Autodesk Fusion 360 part; units mm, degrees
(part 21 of 40)
  line L2220 (15.7293, 63.975) -> (15.8242, 64.105) construction
  line L2221 (15.8242, 64.105) -> (15.92, 64.2346) construction
  line L2222 (15.92, 64.2346) -> (16.0168, 64.3638) construction
  line L2223 (16.0168, 64.3638) -> (16.1146, 64.4926) construction
  line L2224 (16.1146, 64.4926) -> (16.2132, 64.6209) construction
  line L2225 (16.2132, 64.6209) -> (16.3127, 64.7488) construction
  line L2226 (16.3127, 64.7488) -> (16.4131, 64.8762) construction
  line L2227 (16.4131, 64.8762) -> (16.5144, 65.0032) construction
  line L2228 (16.5144, 65.0032) -> (16.6166, 65.1298) construction
  line L2229 (16.6166, 65.1298) -> (16.7196, 65.256) construction
  line L2230 (16.7196, 65.256) -> (16.8235, 65.3817) construction
  line L2231 (16.8235, 65.3817) -> (16.9283, 65.507) construction
  line L2232 (16.9283, 65.507) -> (17.0338, 65.6318) construction
  line L2233 (17.0338, 65.6318) -> (17.1402, 65.7562) construction
  line L2234 (17.1402, 65.7562) -> (17.2474, 65.8802) construction
  line L2235 (17.2474, 65.8802) -> (17.3555, 66.0038) construction
  line L2236 (17.3555, 66.0038) -> (17.4643, 66.1269) construction
  line L2237 (17.4643, 66.1269) -> (17.5739, 66.2497) construction
  line L2238 (17.5739, 66.2497) -> (17.6842, 66.3719) construction
  line L2239 (17.6842, 66.3719) -> (17.7954, 66.4938) construction
  line L2240 (17.7954, 66.4938) -> (17.9073, 66.6152) construction
  line L2241 (17.9073, 66.6152) -> (18.02, 66.7362) construction
  line L2242 (18.02, 66.7362) -> (18.1335, 66.8568) construction
  line L2243 (18.1335, 66.8568) -> (18.2477, 66.9769) construction
  line L2244 (18.2477, 66.9769) -> (18.3626, 67.0966) construction
  line L2245 (18.3626, 67.0966) -> (18.4782, 67.2159) construction
  line L2246 (18.4782, 67.2159) -> (18.5946, 67.3347) construction
  line L2247 (18.5946, 67.3347) -> (18.7118, 67.4531) construction
  line L2248 (18.7118, 67.4531) -> (18.8296, 67.5711) construction
  line L2249 (18.8296, 67.5711) -> (18.9481, 67.6887) construction
  line L2250 (18.9481, 67.6887) -> (19.0674, 67.8058) construction
  line L2251 (19.0674, 67.8058) -> (19.1873, 67.9225) construction
  line L2252 (19.1873, 67.9225) -> (19.3079, 68.0388) construction
  line L2253 (19.3079, 68.0388) -> (19.4293, 68.1546) construction
  line L2254 (19.4293, 68.1546) -> (19.5512, 68.27) construction
  line L2255 (19.5512, 68.27) -> (19.6739, 68.385) construction
  line L2256 (19.6739, 68.385) -> (19.7726, 68.4767) construction
  line L2257 (19.7726, 68.4767) -> (19.8469, 68.5452) construction
  line L2258 (19.8469, 68.5452) -> (19.8966, 68.5908) construction
  line L2259 (19.8966, 68.5908) -> (19.9215, 68.6136) construction
  line L2260 (-24.1948, -56.0345) -> (-24.2071, -56.0628) construction
  line L2261 (-24.2071, -56.0628) -> (-24.2308, -56.1198) construction
  line L2262 (-24.2308, -56.1198) -> (-24.264, -56.2062) construction
  line L2263 (-24.264, -56.2062) -> (-24.3039, -56.3229) construction
  line L2264 (-24.3039, -56.3229) -> (-24.3478, -56.4711) construction
  line L2265 (-24.3478, -56.4711) -> (-24.3873, -56.6208) construction
  line L2266 (-24.3873, -56.6208) -> (-24.4241, -56.7714) construction
  line L2267 (-24.4241, -56.7714) -> (-24.4595, -56.9226) construction
  line L2268 (-24.4595, -56.9226) -> (-24.494, -57.0741) construction
  line L2269 (-24.494, -57.0741) -> (-24.5274, -57.226) construction
  line L2270 (-24.5274, -57.226) -> (-24.5594, -57.3783) construction
  line L2271 (-24.5594, -57.3783) -> (-24.5896, -57.5312) construction
  line L2272 (-24.5896, -57.5312) -> (-24.6176, -57.6848) construction
  line L2273 (-24.6176, -57.6848) -> (-24.6435, -57.8391) construction
  line L2274 (-24.6435, -57.8391) -> (-24.6674, -57.994) construction
  line L2275 (-24.6674, -57.994) -> (-24.6897, -58.1494) construction
  line L2276 (-24.6897, -58.1494) -> (-24.7105, -58.3052) construction
  line L2277 (-24.7105, -58.3052) -> (-24.7301, -58.4614) construction
  line L2278 (-24.7301, -58.4614) -> (-24.7485, -58.6179) construction
  line L2279 (-24.7485, -58.6179) -> (-24.7658, -58.7747) construction
  line L2280 (-24.7658, -58.7747) -> (-24.7818, -58.9318) construction
  line L2281 (-24.7818, -58.9318) -> (-24.7965, -59.0893) construction
  line L2282 (-24.7965, -59.0893) -> (-24.8098, -59.2471) construction
  line L2283 (-24.8098, -59.2471) -> (-24.8218, -59.4053) construction
  line L2284 (-24.8218, -59.4053) -> (-24.8325, -59.5638) construction
  line L2285 (-24.8325, -59.5638) -> (-24.842, -59.7226) construction
  line L2286 (-24.842, -59.7226) -> (-24.8504, -59.8817) construction
  line L2287 (-24.8504, -59.8817) -> (-24.8577, -60.0411) construction
  line L2288 (-24.8577, -60.0411) -> (-24.8638, -60.2007) construction
  line L2289 (-24.8638, -60.2007) -> (-24.8689, -60.3605) construction
  line L2290 (-24.8689, -60.3605) -> (-24.8729, -60.5206) construction
  line L2291 (-24.8729, -60.5206) -> (-24.8757, -60.6809) construction
  line L2292 (-24.8757, -60.6809) -> (-24.8776, -60.8415) construction
  line L2293 (-24.8776, -60.8415) -> (-24.8783, -61.0023) construction
  line L2294 (-24.8783, -61.0023) -> (-24.878, -61.1633) construction
  line L2295 (-24.878, -61.1633) -> (-24.8766, -61.3245) construction
  line L2296 (-24.8766, -61.3245) -> (-24.8742, -61.4859) construction
  line L2297 (-24.8742, -61.4859) -> (-24.8708, -61.6475) construction
  line L2298 (-24.8708, -61.6475) -> (-24.8665, -61.8093) construction
  line L2299 (-24.8665, -61.8093) -> (-24.8611, -61.9712) construction
  line L2300 (-24.8611, -61.9712) -> (-24.8548, -62.1334) construction
  line L2301 (-24.8548, -62.1334) -> (-24.8475, -62.2957) construction
  line L2302 (-24.8475, -62.2957) -> (-24.8392, -62.4581) construction
  line L2303 (-24.8392, -62.4581) -> (-24.83, -62.6207) construction
  line L2304 (-24.83, -62.6207) -> (-24.8199, -62.7835) construction
  line L2305 (-24.8199, -62.7835) -> (-24.8088, -62.9464) construction
  line L2306 (-24.8088, -62.9464) -> (-24.7967, -63.1095) construction
  line L2307 (-24.7967, -63.1095) -> (-24.7838, -63.2727) construction
  line L2308 (-24.7838, -63.2727) -> (-24.77, -63.436) construction
  line L2309 (-24.77, -63.436) -> (-24.7552, -63.5995) construction
  line L2310 (-24.7552, -63.5995) -> (-24.7396, -63.7631) construction
  line L2311 (-24.7396, -63.7631) -> (-24.723, -63.9268) construction
  line L2312 (-24.723, -63.9268) -> (-24.7056, -64.0906) construction
  line L2313 (-24.7056, -64.0906) -> (-24.6873, -64.2545) construction
  line L2314 (-24.6873, -64.2545) -> (-24.6681, -64.4185) construction
  line L2315 (-24.6681, -64.4185) -> (-24.648, -64.5826) construction
  line L2316 (-24.648, -64.5826) -> (-24.6271, -64.7468) construction
  line L2317 (-24.6271, -64.7468) -> (-24.6054, -64.9111) construction
  line L2318 (-24.6054, -64.9111) -> (-24.5828, -65.0755) construction
  line L2319 (-24.5828, -65.0755) -> (-24.5593, -65.24) construction
  line L2320 (-24.5593, -65.24) -> (-24.535, -65.4046) construction
  line L2321 (-24.535, -65.4046) -> (-24.5098, -65.5692) construction
  line L2322 (-24.5098, -65.5692) -> (-24.4839, -65.734) construction
  line L2323 (-24.4839, -65.734) -> (-24.4571, -65.8987) construction
  line L2324 (-24.4571, -65.8987) -> (-24.4294, -66.0636) construction
  line L2325 (-24.4294, -66.0636) -> (-24.401, -66.2285) construction
  line L2326 (-24.401, -66.2285) -> (-24.3718, -66.3935) construction
  line L2327 (-24.3718, -66.3935) -> (-24.3417, -66.5585) construction
  line L2328 (-24.3417, -66.5585) -> (-24.3108, -66.7236) construction
  line L2329 (-24.3108, -66.7236) -> (-24.2792, -66.8887) construction
  line L2330 (-24.2792, -66.8887) -> (-24.2532, -67.0208) construction
  line L2331 (-24.2532, -67.0208) -> (-24.2334, -67.1199) construction
  line L2332 (-24.2334, -67.1199) -> (-24.22, -67.186) construction
  line L2333 (-24.22, -67.186) -> (-24.2132, -67.2191) construction
  line L2334 (-40.3263, -45.8153) -> (-40.3467, -45.8385) construction
  line L2335 (-40.3467, -45.8385) -> (-40.3868, -45.8854) construction
  line L2336 (-40.3868, -45.8854) -> (-40.4451, -45.9573) construction
  line L2337 (-40.4451, -45.9573) -> (-40.5192, -46.056) construction
  line L2338 (-40.5192, -46.056) -> (-40.6066, -46.1833) construction
  line L2339 (-40.6066, -46.1833) -> (-40.6904, -46.3135) construction
  line L2340 (-40.6904, -46.3135) -> (-40.772, -46.4454) construction
  line L2341 (-40.772, -46.4454) -> (-40.8524, -46.5782) construction
  line L2342 (-40.8524, -46.5782) -> (-40.932, -46.7117) construction
  line L2343 (-40.932, -46.7117) -> (-41.0107, -46.8458) construction
  line L2344 (-41.0107, -46.8458) -> (-41.0883, -46.9807) construction
  line L2345 (-41.0883, -46.9807) -> (-41.1642, -47.1168) construction
  line L2346 (-41.1642, -47.1168) -> (-41.2383, -47.2543) construction
  line L2347 (-41.2383, -47.2543) -> (-41.3106, -47.393) construction
  line L2348 (-41.3106, -47.393) -> (-41.3813, -47.5329) construction
  line L2349 (-41.3813, -47.5329) -> (-41.4504, -47.6738) construction
  line L2350 (-41.4504, -47.6738) -> (-41.5184, -47.8156) construction
  line L2351 (-41.5184, -47.8156) -> (-41.5853, -47.9581) construction
  line L2352 (-41.5853, -47.9581) -> (-41.6512, -48.1012) construction
  line L2353 (-41.6512, -48.1012) -> (-41.716, -48.245) construction
  line L2354 (-41.716, -48.245) -> (-41.7798, -48.3895) construction
  line L2355 (-41.7798, -48.3895) -> (-41.8424, -48.5347) construction
  line L2356 (-41.8424, -48.5347) -> (-41.9039, -48.6807) construction
  line L2357 (-41.9039, -48.6807) -> (-41.9642, -48.8274) construction
  line L2358 (-41.9642, -48.8274) -> (-42.0234, -48.9749) construction
  line L2359 (-42.0234, -48.9749) -> (-42.0815, -49.123) construction
  line L2360 (-42.0815, -49.123) -> (-42.1386, -49.2717) construction
  line L2361 (-42.1386, -49.2717) -> (-42.1947, -49.421) construction
  line L2362 (-42.1947, -49.421) -> (-42.2499, -49.5709) construction
  line L2363 (-42.2499, -49.5709) -> (-42.3041, -49.7214) construction
  line L2364 (-42.3041, -49.7214) -> (-42.3574, -49.8724) construction
  line L2365 (-42.3574, -49.8724) -> (-42.4097, -50.024) construction
  line L2366 (-42.4097, -50.024) -> (-42.461, -50.1761) construction
  line L2367 (-42.461, -50.1761) -> (-42.5114, -50.3288) construction
  line L2368 (-42.5114, -50.3288) -> (-42.5608, -50.482) construction
  line L2369 (-42.5608, -50.482) -> (-42.6094, -50.6358) construction
  line L2370 (-42.6094, -50.6358) -> (-42.657, -50.79) construction
  line L2371 (-42.657, -50.79) -> (-42.7037, -50.9447) construction
  line L2372 (-42.7037, -50.9447) -> (-42.7495, -51.0999) construction
  line L2373 (-42.7495, -51.0999) -> (-42.7945, -51.2556) construction
  line L2374 (-42.7945, -51.2556) -> (-42.8386, -51.4118) construction
  line L2375 (-42.8386, -51.4118) -> (-42.8818, -51.5684) construction
  line L2376 (-42.8818, -51.5684) -> (-42.9241, -51.7255) construction
  line L2377 (-42.9241, -51.7255) -> (-42.9656, -51.883) construction
  line L2378 (-42.9656, -51.883) -> (-43.0063, -52.0409) construction
  line L2379 (-43.0063, -52.0409) -> (-43.0461, -52.1993) construction
  line L2380 (-43.0461, -52.1993) -> (-43.085, -52.3581) construction
  line L2381 (-43.085, -52.3581) -> (-43.1231, -52.5173) construction
  line L2382 (-43.1231, -52.5173) -> (-43.1604, -52.6769) construction
  line L2383 (-43.1604, -52.6769) -> (-43.1969, -52.8369) construction
  line L2384 (-43.1969, -52.8369) -> (-43.2326, -52.9973) construction
  line L2385 (-43.2326, -52.9973) -> (-43.2674, -53.1581) construction
  line L2386 (-43.2674, -53.1581) -> (-43.3015, -53.3193) construction
  line L2387 (-43.3015, -53.3193) -> (-43.3347, -53.4809) construction
  line L2388 (-43.3347, -53.4809) -> (-43.3672, -53.6428) construction
  line L2389 (-43.3672, -53.6428) -> (-43.3988, -53.8051) construction
  line L2390 (-43.3988, -53.8051) -> (-43.4297, -53.9677) construction
  line L2391 (-43.4297, -53.9677) -> (-43.4597, -54.1307) construction
  line L2392 (-43.4597, -54.1307) -> (-43.489, -54.294) construction
  line L2393 (-43.489, -54.294) -> (-43.5175, -54.4577) construction
  line L2394 (-43.5175, -54.4577) -> (-43.5453, -54.6217) construction
  line L2395 (-43.5453, -54.6217) -> (-43.5723, -54.7861) construction
  line L2396 (-43.5723, -54.7861) -> (-43.5984, -54.9508) construction
  line L2397 (-43.5984, -54.9508) -> (-43.6239, -55.1158) construction
  line L2398 (-43.6239, -55.1158) -> (-43.6486, -55.2811) construction
  line L2399 (-43.6486, -55.2811) -> (-43.6725, -55.4467) construction
  line L2400 (-43.6725, -55.4467) -> (-43.6956, -55.6126) construction
  line L2401 (-43.6956, -55.6126) -> (-43.718, -55.7789) construction
  line L2402 (-43.718, -55.7789) -> (-43.7397, -55.9454) construction
  line L2403 (-43.7397, -55.9454) -> (-43.7606, -56.1122) construction
  line L2404 (-43.7606, -56.1122) -> (-43.7767, -56.2459) construction
  line L2405 (-43.7767, -56.2459) -> (-43.7885, -56.3463) construction
  line L2406 (-43.7885, -56.3463) -> (-43.7962, -56.4133) construction
  line L2407 (-43.7962, -56.4133) -> (-43.8, -56.4469) construction
  line L2408 (-59.5542, 13.3622) -> (-59.5843, 13.369) construction
  line L2409 (-59.5843, 13.369) -> (-59.6444, 13.3833) construction
  line L2410 (-59.6444, 13.3833) -> (-59.7338, 13.4071) construction
  line L2411 (-59.7338, 13.4071) -> (-59.8517, 13.4435) construction
  line L2412 (-59.8517, 13.4435) -> (-59.9973, 13.4951) construction
  line L2413 (-59.9973, 13.4951) -> (-60.1416, 13.5511) construction
  line L2414 (-60.1416, 13.5511) -> (-60.2852, 13.6099) construction
  line L2415 (-60.2852, 13.6099) -> (-60.4283, 13.6701) construction
  line L2416 (-60.4283, 13.6701) -> (-60.5711, 13.7313) construction
  line L2417 (-60.5711, 13.7313) -> (-60.7136, 13.7935) construction
  line L2418 (-60.7136, 13.7935) -> (-60.8557, 13.8571) construction
  line L2419 (-60.8557, 13.8571) -> (-60.9971, 13.9226) construction
  line L2420 (-60.9971, 13.9226) -> (-61.1379, 13.9902) construction
  line L2421 (-61.1379, 13.9902) -> (-61.2779, 14.06) construction
  line L2422 (-61.2779, 14.06) -> (-61.4173, 14.1316) construction
  line L2423 (-61.4173, 14.1316) -> (-61.5561, 14.205) construction
  line L2424 (-61.5561, 14.205) -> (-61.6944, 14.2797) construction
  line L2425 (-61.6944, 14.2797) -> (-61.8322, 14.3557) construction
  line L2426 (-61.8322, 14.3557) -> (-61.9697, 14.4327) construction
  line L2427 (-61.9697, 14.4327) -> (-62.1067, 14.5109) construction
  line L2428 (-62.1067, 14.5109) -> (-62.2432, 14.5904) construction
  line L2429 (-62.2432, 14.5904) -> (-62.3792, 14.6711) construction
  line L2430 (-62.3792, 14.6711) -> (-62.5148, 14.753) construction
  line L2431 (-62.5148, 14.753) -> (-62.6498, 14.8363) construction
  line L2432 (-62.6498, 14.8363) -> (-62.7843, 14.9208) construction
  line L2433 (-62.7843, 14.9208) -> (-62.9184, 15.0064) construction
  line L2434 (-62.9184, 15.0064) -> (-63.052, 15.0932) construction
  line L2435 (-63.052, 15.0932) -> (-63.1852, 15.181) construction
  line L2436 (-63.1852, 15.181) -> (-63.318, 15.2698) construction
  line L2437 (-63.318, 15.2698) -> (-63.4503, 15.3597) construction
  line L2438 (-63.4503, 15.3597) -> (-63.5821, 15.4506) construction
  line L2439 (-63.5821, 15.4506) -> (-63.7135, 15.5425) construction
  line L2440 (-63.7135, 15.5425) -> (-63.8445, 15.6354) construction
  line L2441 (-63.8445, 15.6354) -> (-63.975, 15.7293) construction
  line L2442 (-63.975, 15.7293) -> (-64.105, 15.8242) construction
  line L2443 (-64.105, 15.8242) -> (-64.2346, 15.92) construction
  line L2444 (-64.2346, 15.92) -> (-64.3638, 16.0168) construction
  line L2445 (-64.3638, 16.0168) -> (-64.4926, 16.1146) construction
  line L2446 (-64.4926, 16.1146) -> (-64.6209, 16.2132) construction
  line L2447 (-64.6209, 16.2132) -> (-64.7488, 16.3127) construction
  line L2448 (-64.7488, 16.3127) -> (-64.8762, 16.4131) construction
  line L2449 (-64.8762, 16.4131) -> (-65.0032, 16.5144) construction
  line L2450 (-65.0032, 16.5144) -> (-65.1298, 16.6166) construction
  line L2451 (-65.1298, 16.6166) -> (-65.256, 16.7196) construction
  line L2452 (-65.256, 16.7196) -> (-65.3817, 16.8235) construction
  line L2453 (-65.3817, 16.8235) -> (-65.507, 16.9283) construction
  line L2454 (-65.507, 16.9283) -> (-65.6318, 17.0338) construction
  line L2455 (-65.6318, 17.0338) -> (-65.7562, 17.1402) construction
  line L2456 (-65.7562, 17.1402) -> (-65.8802, 17.2474) construction
  line L2457 (-65.8802, 17.2474) -> (-66.0038, 17.3555) construction
  line L2458 (-66.0038, 17.3555) -> (-66.1269, 17.4643) construction
  line L2459 (-66.1269, 17.4643) -> (-66.2497, 17.5739) construction
  line L2460 (-66.2497, 17.5739) -> (-66.3719, 17.6842) construction
  line L2461 (-66.3719, 17.6842) -> (-66.4938, 17.7954) construction
  line L2462 (-66.4938, 17.7954) -> (-66.6152, 17.9073) construction
  line L2463 (-66.6152, 17.9073) -> (-66.7362, 18.02) construction
  line L2464 (-66.7362, 18.02) -> (-66.8568, 18.1335) construction
  line L2465 (-66.8568, 18.1335) -> (-66.9769, 18.2477) construction
  line L2466 (-66.9769, 18.2477) -> (-67.0966, 18.3626) construction
  line L2467 (-67.0966, 18.3626) -> (-67.2159, 18.4782) construction
  line L2468 (-67.2159, 18.4782) -> (-67.3347, 18.5946) construction
  line L2469 (-67.3347, 18.5946) -> (-67.4531, 18.7118) construction
  line L2470 (-67.4531, 18.7118) -> (-67.5711, 18.8296) construction
  line L2471 (-67.5711, 18.8296) -> (-67.6887, 18.9481) construction
  line L2472 (-67.6887, 18.9481) -> (-67.8058, 19.0674) construction
  line L2473 (-67.8058, 19.0674) -> (-67.9225, 19.1873) construction
  line L2474 (-67.9225, 19.1873) -> (-68.0388, 19.3079) construction
  line L2475 (-68.0388, 19.3079) -> (-68.1546, 19.4293) construction
  line L2476 (-68.1546, 19.4293) -> (-68.27, 19.5512) construction
  line L2477 (-68.27, 19.5512) -> (-68.385, 19.6739) construction
  line L2478 (-68.385, 19.6739) -> (-68.4767, 19.7726) construction
  line L2479 (-68.4767, 19.7726) -> (-68.5452, 19.8469) construction
  line L2480 (-68.5452, 19.8469) -> (-68.5908, 19.8966) construction
  line L2481 (-68.5908, 19.8966) -> (-68.6136, 19.9215) construction
  line L2482 (-31.1115, 52.5103) -> (-31.1272, 52.5368) construction
  line L2483 (-31.1272, 52.5368) -> (-31.1594, 52.5895) construction
  line L2484 (-31.1594, 52.5895) -> (-31.2097, 52.6672) construction
  line L2485 (-31.2097, 52.6672) -> (-31.2807, 52.7681) construction
  line L2486 (-31.2807, 52.7681) -> (-31.3748, 52.8906) construction
  line L2487 (-31.3748, 52.8906) -> (-31.4727, 53.0106) construction
  line L2488 (-31.4727, 53.0106) -> (-31.5729, 53.1289) construction
  line L2489 (-31.5729, 53.1289) -> (-31.6744, 53.2464) construction
  line L2490 (-31.6744, 53.2464) -> (-31.7767, 53.3634) construction
  line L2491 (-31.7767, 53.3634) -> (-31.88, 53.4797) construction
  line L2492 (-31.88, 53.4797) -> (-31.9844, 53.5951) construction
  line L2493 (-31.9844, 53.5951) -> (-32.0903, 53.7094) construction
  line L2494 (-32.0903, 53.7094) -> (-32.1981, 53.8224) construction
  line L2495 (-32.1981, 53.8224) -> (-32.3077, 53.934) construction
  line L2496 (-32.3077, 53.934) -> (-32.419, 54.0444) construction
  line L2497 (-32.419, 54.0444) -> (-32.5316, 54.1537) construction
  line L2498 (-32.5316, 54.1537) -> (-32.6455, 54.2622) construction
  line L2499 (-32.6455, 54.2622) -> (-32.7603, 54.3698) construction
  line L2500 (-32.7603, 54.3698) -> (-32.876, 54.4767) construction
  line L2501 (-32.876, 54.4767) -> (-32.9927, 54.5828) construction
  line L2502 (-32.9927, 54.5828) -> (-33.1105, 54.6881) construction
  line L2503 (-33.1105, 54.6881) -> (-33.2292, 54.7926) construction
  line L2504 (-33.2292, 54.7926) -> (-33.3491, 54.8961) construction
  line L2505 (-33.3491, 54.8961) -> (-33.47, 54.9988) construction
  line L2506 (-33.47, 54.9988) -> (-33.5919, 55.1007) construction
  line L2507 (-33.5919, 55.1007) -> (-33.7148, 55.2017) construction
  line L2508 (-33.7148, 55.2017) -> (-33.8386, 55.302) construction
  line L2509 (-33.8386, 55.302) -> (-33.9633, 55.4015) construction
  line L2510 (-33.9633, 55.4015) -> (-34.0888, 55.5003) construction
  line L2511 (-34.0888, 55.5003) -> (-34.2151, 55.5984) construction
  line L2512 (-34.2151, 55.5984) -> (-34.3423, 55.6957) construction
  line L2513 (-34.3423, 55.6957) -> (-34.4703, 55.7923) construction
  line L2514 (-34.4703, 55.7923) -> (-34.5991, 55.8881) construction
  line L2515 (-34.5991, 55.8881) -> (-34.7288, 55.9832) construction
  line L2516 (-34.7288, 55.9832) -> (-34.8592, 56.0776) construction
  line L2517 (-34.8592, 56.0776) -> (-34.9905, 56.1712) construction
  line L2518 (-34.9905, 56.1712) -> (-35.1224, 56.2642) construction
  line L2519 (-35.1224, 56.2642) -> (-35.2552, 56.3564) construction
  line L2520 (-35.2552, 56.3564) -> (-35.3886, 56.448) construction
  line L2521 (-35.3886, 56.448) -> (-35.5228, 56.5388) construction
  line L2522 (-35.5228, 56.5388) -> (-35.6577, 56.629) construction
  line L2523 (-35.6577, 56.629) -> (-35.7933, 56.7185) construction
  line L2524 (-35.7933, 56.7185) -> (-35.9295, 56.8073) construction
  line L2525 (-35.9295, 56.8073) -> (-36.0665, 56.8955) construction
  line L2526 (-36.0665, 56.8955) -> (-36.2042, 56.9829) construction
  line L2527 (-36.2042, 56.9829) -> (-36.3425, 57.0697) construction
  line L2528 (-36.3425, 57.0697) -> (-36.4815, 57.1558) construction
  line L2529 (-36.4815, 57.1558) -> (-36.6211, 57.2413) construction
  line L2530 (-36.6211, 57.2413) -> (-36.7614, 57.3261) construction
  line L2531 (-36.7614, 57.3261) -> (-36.9023, 57.4102) construction
  line L2532 (-36.9023, 57.4102) -> (-37.0438, 57.4937) construction
  line L2533 (-37.0438, 57.4937) -> (-37.186, 57.5765) construction
  line L2534 (-37.186, 57.5765) -> (-37.3288, 57.6587) construction
  line L2535 (-37.3288, 57.6587) -> (-37.4721, 57.7403) construction
  line L2536 (-37.4721, 57.7403) -> (-37.6161, 57.8212) construction
  line L2537 (-37.6161, 57.8212) -> (-37.7607, 57.9014) construction
  line L2538 (-37.7607, 57.9014) -> (-37.9058, 57.981) construction
  line L2539 (-37.9058, 57.981) -> (-38.0515, 58.06) construction
  line L2540 (-38.0515, 58.06) -> (-38.1978, 58.1383) construction
  line L2541 (-38.1978, 58.1383) -> (-38.3447, 58.216) construction
  line L2542 (-38.3447, 58.216) -> (-38.4921, 58.2931) construction
  line L2543 (-38.4921, 58.2931) -> (-38.6401, 58.3695) construction
  line L2544 (-38.6401, 58.3695) -> (-38.7886, 58.4453) construction
  line L2545 (-38.7886, 58.4453) -> (-38.9377, 58.5205) construction
  line L2546 (-38.9377, 58.5205) -> (-39.0873, 58.595) construction
  line L2547 (-39.0873, 58.595) -> (-39.2374, 58.669) construction
  line L2548 (-39.2374, 58.669) -> (-39.3881, 58.7423) construction
  line L2549 (-39.3881, 58.7423) -> (-39.5393, 58.8149) construction
  line L2550 (-39.5393, 58.8149) -> (-39.6909, 58.887) construction
  line L2551 (-39.6909, 58.887) -> (-39.8431, 58.9584) construction
  line L2552 (-39.8431, 58.9584) -> (-39.9653, 59.0151) construction
  line L2553 (-39.9653, 59.0151) -> (-40.0572, 59.0573) construction
  line L2554 (-40.0572, 59.0573) -> (-40.1185, 59.0853) construction
  line L2555 (-40.1185, 59.0853) -> (-40.1492, 59.0993) construction
  line L2556 (52.5103, 31.1115) -> (52.5368, 31.1272) construction
  line L2557 (52.5368, 31.1272) -> (52.5895, 31.1594) construction
  line L2558 (52.5895, 31.1594) -> (52.6672, 31.2097) construction
  line L2559 (52.6672, 31.2097) -> (52.7681, 31.2807) construction
  line L2560 (52.7681, 31.2807) -> (52.8906, 31.3748) construction
  line L2561 (52.8906, 31.3748) -> (53.0106, 31.4727) construction
  line L2562 (53.0106, 31.4727) -> (53.1289, 31.5729) construction
  line L2563 (53.1289, 31.5729) -> (53.2464, 31.6744) construction
  line L2564 (53.2464, 31.6744) -> (53.3634, 31.7767) construction
  line L2565 (53.3634, 31.7767) -> (53.4797, 31.88) construction
  line L2566 (53.4797, 31.88) -> (53.5951, 31.9844) construction
  line L2567 (53.5951, 31.9844) -> (53.7094, 32.0903) construction
  line L2568 (53.7094, 32.0903) -> (53.8224, 32.1981) construction
  line L2569 (53.8224, 32.1981) -> (53.934, 32.3077) construction
  line L2570 (53.934, 32.3077) -> (54.0444, 32.419) construction
  line L2571 (54.0444, 32.419) -> (54.1537, 32.5316) construction
  line L2572 (54.1537, 32.5316) -> (54.2622, 32.6455) construction
  line L2573 (54.2622, 32.6455) -> (54.3698, 32.7603) construction
  line L2574 (54.3698, 32.7603) -> (54.4767, 32.876) construction
  line L2575 (54.4767, 32.876) -> (54.5828, 32.9927) construction
  line L2576 (54.5828, 32.9927) -> (54.6881, 33.1105) construction
  line L2577 (54.6881, 33.1105) -> (54.7926, 33.2292) construction
  line L2578 (54.7926, 33.2292) -> (54.8961, 33.3491) construction
  line L2579 (54.8961, 33.3491) -> (54.9988, 33.47) construction
  line L2580 (54.9988, 33.47) -> (55.1007, 33.5919) construction
  line L2581 (55.1007, 33.5919) -> (55.2017, 33.7148) construction
  line L2582 (55.2017, 33.7148) -> (55.302, 33.8386) construction
  line L2583 (55.302, 33.8386) -> (55.4015, 33.9633) construction
  line L2584 (55.4015, 33.9633) -> (55.5003, 34.0888) construction
  line L2585 (55.5003, 34.0888) -> (55.5984, 34.2151) construction
  line L2586 (55.5984, 34.2151) -> (55.6957, 34.3423) construction
  line L2587 (55.6957, 34.3423) -> (55.7923, 34.4703) construction
  line L2588 (55.7923, 34.4703) -> (55.8881, 34.5991) construction
  line L2589 (55.8881, 34.5991) -> (55.9832, 34.7288) construction
  line L2590 (55.9832, 34.7288) -> (56.0776, 34.8592) construction
  line L2591 (56.0776, 34.8592) -> (56.1712, 34.9905) construction
  line L2592 (56.1712, 34.9905) -> (56.2642, 35.1224) construction
  line L2593 (56.2642, 35.1224) -> (56.3564, 35.2552) construction
  line L2594 (56.3564, 35.2552) -> (56.448, 35.3886) construction
  line L2595 (56.448, 35.3886) -> (56.5388, 35.5228) construction
  line L2596 (56.5388, 35.5228) -> (56.629, 35.6577) construction
  line L2597 (56.629, 35.6577) -> (56.7185, 35.7933) construction
  line L2598 (56.7185, 35.7933) -> (56.8073, 35.9295) construction
  line L2599 (56.8073, 35.9295) -> (56.8955, 36.0665) construction
  line L2600 (56.8955, 36.0665) -> (56.9829, 36.2042) construction
  line L2601 (56.9829, 36.2042) -> (57.0697, 36.3425) construction
  line L2602 (57.0697, 36.3425) -> (57.1558, 36.4815) construction
  line L2603 (57.1558, 36.4815) -> (57.2413, 36.6211) construction
  line L2604 (57.2413, 36.6211) -> (57.3261, 36.7614) construction
  line L2605 (57.3261, 36.7614) -> (57.4102, 36.9023) construction
  line L2606 (57.4102, 36.9023) -> (57.4937, 37.0438) construction
  line L2607 (57.4937, 37.0438) -> (57.5765, 37.186) construction
  line L2608 (57.5765, 37.186) -> (57.6587, 37.3288) construction
  line L2609 (57.6587, 37.3288) -> (57.7403, 37.4721) construction
  line L2610 (57.7403, 37.4721) -> (57.8212, 37.6161) construction
  line L2611 (57.8212, 37.6161) -> (57.9014, 37.7607) construction
  line L2612 (57.9014, 37.7607) -> (57.981, 37.9058) construction
  line L2613 (57.981, 37.9058) -> (58.06, 38.0515) construction
  line L2614 (58.06, 38.0515) -> (58.1383, 38.1978) construction
  line L2615 (58.1383, 38.1978) -> (58.216, 38.3447) construction
  line L2616 (58.216, 38.3447) -> (58.2931, 38.4921) construction
  line L2617 (58.2931, 38.4921) -> (58.3695, 38.6401) construction
  line L2618 (58.3695, 38.6401) -> (58.4453, 38.7886) construction
  line L2619 (58.4453, 38.7886) -> (58.5205, 38.9377) construction
  line L2620 (58.5205, 38.9377) -> (58.595, 39.0873) construction
  line L2621 (58.595, 39.0873) -> (58.669, 39.2374) construction
  line L2622 (58.669, 39.2374) -> (58.7423, 39.3881) construction
  line L2623 (58.7423, 39.3881) -> (58.8149, 39.5393) construction
  line L2624 (58.8149, 39.5393) -> (58.887, 39.6909) construction
  line L2625 (58.887, 39.6909) -> (58.9584, 39.8431) construction
  line L2626 (58.9584, 39.8431) -> (59.0151, 39.9653) construction
  line L2627 (59.0151, 39.9653) -> (59.0573, 40.0572) construction
  line L2628 (59.0573, 40.0572) -> (59.0853, 40.1185) construction
  line L2629 (59.0853, 40.1185) -> (59.0993, 40.1492) construction
  line L2630 (-40.3263, 45.8153) -> (-40.3467, 45.8385) construction
  line L2631 (-40.3467, 45.8385) -> (-40.3868, 45.8854) construction
  line L2632 (-40.3868, 45.8854) -> (-40.4451, 45.9573) construction
  line L2633 (-40.4451, 45.9573) -> (-40.5192, 46.056) construction
  line L2634 (-40.5192, 46.056) -> (-40.6066, 46.1833) construction
  line L2635 (-40.6066, 46.1833) -> (-40.6904, 46.3135) construction
  line L2636 (-40.6904, 46.3135) -> (-40.772, 46.4454) construction
  line L2637 (-40.772, 46.4454) -> (-40.8524, 46.5782) construction
  line L2638 (-40.8524, 46.5782) -> (-40.932, 46.7117) construction
  line L2639 (-40.932, 46.7117) -> (-41.0107, 46.8458) construction
  line L2640 (-41.0107, 46.8458) -> (-41.0883, 46.9807) construction
  line L2641 (-41.0883, 46.9807) -> (-41.1642, 47.1168) construction
  line L2642 (-41.1642, 47.1168) -> (-41.2383, 47.2543) construction
  line L2643 (-41.2383, 47.2543) -> (-41.3106, 47.393) construction
  line L2644 (-41.3106, 47.393) -> (-41.3813, 47.5329) construction
  line L2645 (-41.3813, 47.5329) -> (-41.4504, 47.6738) construction
  line L2646 (-41.4504, 47.6738) -> (-41.5184, 47.8156) construction
  line L2647 (-41.5184, 47.8156) -> (-41.5853, 47.9581) construction
  line L2648 (-41.5853, 47.9581) -> (-41.6512, 48.1012) construction
  line L2649 (-41.6512, 48.1012) -> (-41.716, 48.245) construction
  line L2650 (-41.716, 48.245) -> (-41.7798, 48.3895) construction
  line L2651 (-41.7798, 48.3895) -> (-41.8424, 48.5347) construction
  line L2652 (-41.8424, 48.5347) -> (-41.9039, 48.6807) construction
  line L2653 (-41.9039, 48.6807) -> (-41.9642, 48.8274) construction
  line L2654 (-41.9642, 48.8274) -> (-42.0234, 48.9749) construction
  line L2655 (-42.0234, 48.9749) -> (-42.0815, 49.123) construction
  line L2656 (-42.0815, 49.123) -> (-42.1386, 49.2717) construction
  line L2657 (-42.1386, 49.2717) -> (-42.1947, 49.421) construction
  line L2658 (-42.1947, 49.421) -> (-42.2499, 49.5709) construction
  line L2659 (-42.2499, 49.5709) -> (-42.3041, 49.7214) construction
  line L2660 (-42.3041, 49.7214) -> (-42.3574, 49.8724) construction
  line L2661 (-42.3574, 49.8724) -> (-42.4097, 50.024) construction
  line L2662 (-42.4097, 50.024) -> (-42.461, 50.1761) construction
  line L2663 (-42.461, 50.1761) -> (-42.5114, 50.3288) construction
  line L2664 (-42.5114, 50.3288) -> (-42.5608, 50.482) construction
  line L2665 (-42.5608, 50.482) -> (-42.6094, 50.6358) construction
  line L2666 (-42.6094, 50.6358) -> (-42.657, 50.79) construction
  line L2667 (-42.657, 50.79) -> (-42.7037, 50.9447) construction
  line L2668 (-42.7037, 50.9447) -> (-42.7495, 51.0999) construction
  line L2669 (-42.7495, 51.0999) -> (-42.7945, 51.2556) construction
  line L2670 (-42.7945, 51.2556) -> (-42.8386, 51.4118) construction
  line L2671 (-42.8386, 51.4118) -> (-42.8818, 51.5684) construction
  line L2672 (-42.8818, 51.5684) -> (-42.9241, 51.7255) construction
  line L2673 (-42.9241, 51.7255) -> (-42.9656, 51.883) construction
  line L2674 (-42.9656, 51.883) -> (-43.0063, 52.0409) construction
  line L2675 (-43.0063, 52.0409) -> (-43.0461, 52.1993) construction
  line L2676 (-43.0461, 52.1993) -> (-43.085, 52.3581) construction
  line L2677 (-43.085, 52.3581) -> (-43.1231, 52.5173) construction
  line L2678 (-43.1231, 52.5173) -> (-43.1604, 52.6769) construction
  line L2679 (-43.1604, 52.6769) -> (-43.1969, 52.8369) construction
  line L2680 (-43.1969, 52.8369) -> (-43.2326, 52.9973) construction
  line L2681 (-43.2326, 52.9973) -> (-43.2674, 53.1581) construction
  line L2682 (-43.2674, 53.1581) -> (-43.3015, 53.3193) construction
  line L2683 (-43.3015, 53.3193) -> (-43.3347, 53.4809) construction
  line L2684 (-43.3347, 53.4809) -> (-43.3672, 53.6428) construction
  line L2685 (-43.3672, 53.6428) -> (-43.3988, 53.8051) construction
  line L2686 (-43.3988, 53.8051) -> (-43.4297, 53.9677) construction
  line L2687 (-43.4297, 53.9677) -> (-43.4597, 54.1307) construction
  line L2688 (-43.4597, 54.1307) -> (-43.489, 54.294) construction
  line L2689 (-43.489, 54.294) -> (-43.5175, 54.4577) construction
  line L2690 (-43.5175, 54.4577) -> (-43.5453, 54.6217) construction
  line L2691 (-43.5453, 54.6217) -> (-43.5723, 54.7861) construction
  line L2692 (-43.5723, 54.7861) -> (-43.5984, 54.9508) construction
  line L2693 (-43.5984, 54.9508) -> (-43.6239, 55.1158) construction
  line L2694 (-43.6239, 55.1158) -> (-43.6486, 55.2811) construction
  line L2695 (-43.6486, 55.2811) -> (-43.6725, 55.4467) construction
  line L2696 (-43.6725, 55.4467) -> (-43.6956, 55.6126) construction
  line L2697 (-43.6956, 55.6126) -> (-43.718, 55.7789) construction
  line L2698 (-43.718, 55.7789) -> (-43.7397, 55.9454) construction
  line L2699 (-43.7397, 55.9454) -> (-43.7606, 56.1122) construction
  line L2700 (-43.7606, 56.1122) -> (-43.7767, 56.2459) construction
  line L2701 (-43.7767, 56.2459) -> (-43.7885, 56.3463) construction
  line L2702 (-43.7885, 56.3463) -> (-43.7962, 56.4133) construction
  line L2703 (-43.7962, 56.4133) -> (-43.8, 56.4469) construction
  line L2704 (-56.0345, 24.1948) -> (-56.0628, 24.2071) construction
  line L2705 (-56.0628, 24.2071) -> (-56.1198, 24.2308) construction
  line L2706 (-56.1198, 24.2308) -> (-56.2062, 24.264) construction
  line L2707 (-56.2062, 24.264) -> (-56.3229, 24.3039) construction
  line L2708 (-56.3229, 24.3039) -> (-56.4711, 24.3478) construction
  line L2709 (-56.4711, 24.3478) -> (-56.6208, 24.3873) construction
  line L2710 (-56.6208, 24.3873) -> (-56.7714, 24.4241) construction
  line L2711 (-56.7714, 24.4241) -> (-56.9226, 24.4595) construction
  line L2712 (-56.9226, 24.4595) -> (-57.0741, 24.494) construction
  line L2713 (-57.0741, 24.494) -> (-57.226, 24.5274) construction
  line L2714 (-57.226, 24.5274) -> (-57.3783, 24.5594) construction
  line L2715 (-57.3783, 24.5594) -> (-57.5312, 24.5896) construction
  line L2716 (-57.5312, 24.5896) -> (-57.6848, 24.6176) construction
  line L2717 (-57.6848, 24.6176) -> (-57.8391, 24.6435) construction
  line L2718 (-57.8391, 24.6435) -> (-57.994, 24.6674) construction
  line L2719 (-57.994, 24.6674) -> (-58.1494, 24.6897) construction
  line L2720 (-58.1494, 24.6897) -> (-58.3052, 24.7105) construction
  line L2721 (-58.3052, 24.7105) -> (-58.4614, 24.7301) construction
  line L2722 (-58.4614, 24.7301) -> (-58.6179, 24.7485) construction
  line L2723 (-58.6179, 24.7485) -> (-58.7747, 24.7658) construction
  line L2724 (-58.7747, 24.7658) -> (-58.9318, 24.7818) construction
  line L2725 (-58.9318, 24.7818) -> (-59.0893, 24.7965) construction
  line L2726 (-59.0893, 24.7965) -> (-59.2471, 24.8098) construction
  line L2727 (-59.2471, 24.8098) -> (-59.4053, 24.8218) construction
  line L2728 (-59.4053, 24.8218) -> (-59.5638, 24.8325) construction
  line L2729 (-59.5638, 24.8325) -> (-59.7226, 24.842) construction
  line L2730 (-59.7226, 24.842) -> (-59.8817, 24.8504) construction
  line L2731 (-59.8817, 24.8504) -> (-60.0411, 24.8577) construction
  line L2732 (-60.0411, 24.8577) -> (-60.2007, 24.8638) construction
  line L2733 (-60.2007, 24.8638) -> (-60.3605, 24.8689) construction
  line L2734 (-60.3605, 24.8689) -> (-60.5206, 24.8729) construction
  line L2735 (-60.5206, 24.8729) -> (-60.6809, 24.8757) construction
  line L2736 (-60.6809, 24.8757) -> (-60.8415, 24.8776) construction
  line L2737 (-60.8415, 24.8776) -> (-61.0023, 24.8783) construction
  line L2738 (-61.0023, 24.8783) -> (-61.1633, 24.878) construction
  line L2739 (-61.1633, 24.878) -> (-61.3245, 24.8766) construction
  line L2740 (-61.3245, 24.8766) -> (-61.4859, 24.8742) construction
  line L2741 (-61.4859, 24.8742) -> (-61.6475, 24.8708) construction
  line L2742 (-61.6475, 24.8708) -> (-61.8093, 24.8665) construction
  line L2743 (-61.8093, 24.8665) -> (-61.9712, 24.8611) construction
  line L2744 (-61.9712, 24.8611) -> (-62.1334, 24.8548) construction
  line L2745 (-62.1334, 24.8548) -> (-62.2957, 24.8475) construction
  line L2746 (-62.2957, 24.8475) -> (-62.4581, 24.8392) construction
  line L2747 (-62.4581, 24.8392) -> (-62.6207, 24.83) construction
  line L2748 (-62.6207, 24.83) -> (-62.7835, 24.8199) construction
  line L2749 (-62.7835, 24.8199) -> (-62.9464, 24.8088) construction
  line L2750 (-62.9464, 24.8088) -> (-63.1095, 24.7967) construction
  line L2751 (-63.1095, 24.7967) -> (-63.2727, 24.7838) construction
  line L2752 (-63.2727, 24.7838) -> (-63.436, 24.77) construction
  line L2753 (-63.436, 24.77) -> (-63.5995, 24.7552) construction
  line L2754 (-63.5995, 24.7552) -> (-63.7631, 24.7396) construction
  line L2755 (-63.7631, 24.7396) -> (-63.9268, 24.723) construction
  line L2756 (-63.9268, 24.723) -> (-64.0906, 24.7056) construction
  line L2757 (-64.0906, 24.7056) -> (-64.2545, 24.6873) construction
  line L2758 (-64.2545, 24.6873) -> (-64.4185, 24.6681) construction
  line L2759 (-64.4185, 24.6681) -> (-64.5826, 24.648) construction
  line L2760 (-64.5826, 24.648) -> (-64.7468, 24.6271) construction
  line L2761 (-64.7468, 24.6271) -> (-64.9111, 24.6054) construction
  line L2762 (-64.9111, 24.6054) -> (-65.0755, 24.5828) construction
  line L2763 (-65.0755, 24.5828) -> (-65.24, 24.5593) construction
  line L2764 (-65.24, 24.5593) -> (-65.4046, 24.535) construction
  line L2765 (-65.4046, 24.535) -> (-65.5692, 24.5098) construction
  line L2766 (-65.5692, 24.5098) -> (-65.734, 24.4839) construction
  line L2767 (-65.734, 24.4839) -> (-65.8987, 24.4571) construction
  line L2768 (-65.8987, 24.4571) -> (-66.0636, 24.4294) construction
  line L2769 (-66.0636, 24.4294) -> (-66.2285, 24.401) construction
  line L2770 (-66.2285, 24.401) -> (-66.3935, 24.3718) construction
  line L2771 (-66.3935, 24.3718) -> (-66.5585, 24.3417) construction
  line L2772 (-66.5585, 24.3417) -> (-66.7236, 24.3108) construction
  line L2773 (-66.7236, 24.3108) -> (-66.8887, 24.2792) construction
  line L2774 (-66.8887, 24.2792) -> (-67.0208, 24.2532) construction
  line L2775 (-67.0208, 24.2532) -> (-67.1199, 24.2334) construction
  line L2776 (-67.1199, 24.2334) -> (-67.186, 24.22) construction
  line L2777 (-67.186, 24.22) -> (-67.2191, 24.2132) construction
  line L2778 (59.5542, -13.3622) -> (59.5843, -13.369) construction
  line L2779 (59.5843, -13.369) -> (59.6444, -13.3833) construction
  line L2780 (59.6444, -13.3833) -> (59.7338, -13.4071) construction
  line L2781 (59.7338, -13.4071) -> (59.8517, -13.4435) construction
  line L2782 (59.8517, -13.4435) -> (59.9973, -13.4951) construction
  line L2783 (59.9973, -13.4951) -> (60.1416, -13.5511) construction
  line L2784 (60.1416, -13.5511) -> (60.2852, -13.6099) construction
  line L2785 (60.2852, -13.6099) -> (60.4283, -13.6701) construction
  line L2786 (60.4283, -13.6701) -> (60.5711, -13.7313) construction
  line L2787 (60.5711, -13.7313) -> (60.7136, -13.7935) construction
  line L2788 (60.7136, -13.7935) -> (60.8557, -13.8571) construction
  line L2789 (60.8557, -13.8571) -> (60.9971, -13.9226) construction
  line L2790 (60.9971, -13.9226) -> (61.1379, -13.9902) construction
  line L2791 (61.1379, -13.9902) -> (61.2779, -14.06) construction
  line L2792 (61.2779, -14.06) -> (61.4173, -14.1316) construction
  line L2793 (61.4173, -14.1316) -> (61.5561, -14.205) construction
  line L2794 (61.5561, -14.205) -> (61.6944, -14.2797) construction
  line L2795 (61.6944, -14.2797) -> (61.8322, -14.3557) construction
  line L2796 (61.8322, -14.3557) -> (61.9697, -14.4327) construction
  line L2797 (61.9697, -14.4327) -> (62.1067, -14.5109) construction
  line L2798 (62.1067, -14.5109) -> (62.2432, -14.5904) construction
  line L2799 (62.2432, -14.5904) -> (62.3792, -14.6711) construction
  line L2800 (62.3792, -14.6711) -> (62.5148, -14.753) construction
  line L2801 (62.5148, -14.753) -> (62.6498, -14.8363) construction
  line L2802 (62.6498, -14.8363) -> (62.7843, -14.9208) construction
  line L2803 (62.7843, -14.9208) -> (62.9184, -15.0064) construction
  line L2804 (62.9184, -15.0064) -> (63.052, -15.0932) construction
  line L2805 (63.052, -15.0932) -> (63.1852, -15.181) construction
  line L2806 (63.1852, -15.181) -> (63.318, -15.2698) construction
  line L2807 (63.318, -15.2698) -> (63.4503, -15.3597) construction
  line L2808 (63.4503, -15.3597) -> (63.5821, -15.4506) construction
  line L2809 (63.5821, -15.4506) -> (63.7135, -15.5425) construction
  line L2810 (63.7135, -15.5425) -> (63.8445, -15.6354) construction
  line L2811 (63.8445, -15.6354) -> (63.975, -15.7293) construction
  line L2812 (63.975, -15.7293) -> (64.105, -15.8242) construction
  line L2813 (64.105, -15.8242) -> (64.2346, -15.92) construction
  line L2814 (64.2346, -15.92) -> (64.3638, -16.0168) construction
  line L2815 (64.3638, -16.0168) -> (64.4926, -16.1146) construction
  line L2816 (64.4926, -16.1146) -> (64.6209, -16.2132) construction
  line L2817 (64.6209, -16.2132) -> (64.7488, -16.3127) construction
  line L2818 (64.7488, -16.3127) -> (64.8762, -16.4131) construction
  line L2819 (64.8762, -16.4131) -> (65.0032, -16.5144) construction
  line L2820 (65.0032, -16.5144) -> (65.1298, -16.6166) construction
  line L2821 (65.1298, -16.6166) -> (65.256, -16.7196) construction
  line L2822 (65.256, -16.7196) -> (65.3817, -16.8235) construction
  line L2823 (65.3817, -16.8235) -> (65.507, -16.9283) construction
  line L2824 (65.507, -16.9283) -> (65.6318, -17.0338) construction
  line L2825 (65.6318, -17.0338) -> (65.7562, -17.1402) construction
  line L2826 (65.7562, -17.1402) -> (65.8802, -17.2474) construction
  line L2827 (65.8802, -17.2474) -> (66.0038, -17.3555) construction
  line L2828 (66.0038, -17.3555) -> (66.1269, -17.4643) construction
  line L2829 (66.1269, -17.4643) -> (66.2497, -17.5739) construction
  line L2830 (66.2497, -17.5739) -> (66.3719, -17.6842) construction
  line L2831 (66.3719, -17.6842) -> (66.4938, -17.7954) construction
  line L2832 (66.4938, -17.7954) -> (66.6152, -17.9073) construction
  line L2833 (66.6152, -17.9073) -> (66.7362, -18.02) construction
  line L2834 (66.7362, -18.02) -> (66.8568, -18.1335) construction
  line L2835 (66.8568, -18.1335) -> (66.9769, -18.2477) construction
  line L2836 (66.9769, -18.2477) -> (67.0966, -18.3626) construction
  line L2837 (67.0966, -18.3626) -> (67.2159, -18.4782) construction
  line L2838 (67.2159, -18.4782) -> (67.3347, -18.5946) construction
  line L2839 (67.3347, -18.5946) -> (67.4531, -18.7118) construction
  line L2840 (67.4531, -18.7118) -> (67.5711, -18.8296) construction
  line L2841 (67.5711, -18.8296) -> (67.6887, -18.9481) construction
  line L2842 (67.6887, -18.9481) -> (67.8058, -19.0674) construction
  line L2843 (67.8058, -19.0674) -> (67.9225, -19.1873) construction
  line L2844 (67.9225, -19.1873) -> (68.0388, -19.3079) construction
  line L2845 (68.0388, -19.3079) -> (68.1546, -19.4293) construction
  line L2846 (68.1546, -19.4293) -> (68.27, -19.5512) construction
  line L2847 (68.27, -19.5512) -> (68.385, -19.6739) construction
  line L2848 (68.385, -19.6739) -> (68.4767, -19.7726) construction
  line L2849 (68.4767, -19.7726) -> (68.5452, -19.8469) construction
  line L2850 (68.5452, -19.8469) -> (68.5908, -19.8966) construction
  line L2851 (68.5908, -19.8966) -> (68.6136, -19.9215) construction
  line L2852 (-60.7685, 5.6951) -> (-60.7993, 5.6979) construction
  line L2853 (-60.7993, 5.6979) -> (-60.8609, 5.7029) construction
  line L2854 (-60.8609, 5.7029) -> (-60.9533, 5.7078) construction
  line L2855 (-60.9533, 5.7078) -> (-61.0766, 5.7097) construction
  line L2856 (-61.0766, 5.7097) -> (-61.231, 5.7056) construction
  line L2857 (-61.231, 5.7056) -> (-61.3856, 5.6969) construction
  line L2858 (-61.3856, 5.6969) -> (-61.5403, 5.6854) construction
  line L2859 (-61.5403, 5.6854) -> (-61.695, 5.6723) construction
  line L2860 (-61.695, 5.6723) -> (-61.8498, 5.6583) construction
  line L2861 (-61.8498, 5.6583) -> (-62.0045, 5.6431) construction
  line L2862 (-62.0045, 5.6431) -> (-62.1593, 5.6265) construction
  line L2863 (-62.1593, 5.6265) -> (-62.314, 5.608) construction
  line L2864 (-62.314, 5.608) -> (-62.4688, 5.5871) construction
  line L2865 (-62.4688, 5.5871) -> (-62.6235, 5.5641) construction
  line L2866 (-62.6235, 5.5641) -> (-62.7782, 5.539) construction
  line L2867 (-62.7782, 5.539) -> (-62.9329, 5.5121) construction
  line L2868 (-62.9329, 5.5121) -> (-63.0875, 5.4838) construction
  line L2869 (-63.0875, 5.4838) -> (-63.2421, 5.4542) construction
  line L2870 (-63.2421, 5.4542) -> (-63.3966, 5.4233) construction
  line L2871 (-63.3966, 5.4233) -> (-63.5511, 5.3913) construction
  line L2872 (-63.5511, 5.3913) -> (-63.7055, 5.3579) construction
  line L2873 (-63.7055, 5.3579) -> (-63.8598, 5.3232) construction
  line L2874 (-63.8598, 5.3232) -> (-64.014, 5.2871) construction
  line L2875 (-64.014, 5.2871) -> (-64.1682, 5.2497) construction
  line L2876 (-64.1682, 5.2497) -> (-64.3222, 5.2109) construction
  line L2877 (-64.3222, 5.2109) -> (-64.4762, 5.1709) construction
  line L2878 (-64.4762, 5.1709) -> (-64.6301, 5.1297) construction
  line L2879 (-64.6301, 5.1297) -> (-64.7839, 5.0873) construction
  line L2880 (-64.7839, 5.0873) -> (-64.9376, 5.0439) construction
  line L2881 (-64.9376, 5.0439) -> (-65.0912, 4.9993) construction
  line L2882 (-65.0912, 4.9993) -> (-65.2447, 4.9536) construction
  line L2883 (-65.2447, 4.9536) -> (-65.398, 4.9068) construction
  line L2884 (-65.398, 4.9068) -> (-65.5513, 4.8589) construction
  line L2885 (-65.5513, 4.8589) -> (-65.7044, 4.8099) construction
  line L2886 (-65.7044, 4.8099) -> (-65.8574, 4.7599) construction
  line L2887 (-65.8574, 4.7599) -> (-66.0103, 4.7087) construction
  line L2888 (-66.0103, 4.7087) -> (-66.1631, 4.6566) construction
  line L2889 (-66.1631, 4.6566) -> (-66.3158, 4.6035) construction
  line L2890 (-66.3158, 4.6035) -> (-66.4683, 4.5493) construction
  line L2891 (-66.4683, 4.5493) -> (-66.6206, 4.4942) construction
  line L2892 (-66.6206, 4.4942) -> (-66.7729, 4.438) construction
  line L2893 (-66.7729, 4.438) -> (-66.925, 4.381) construction
  line L2894 (-66.925, 4.381) -> (-67.077, 4.3229) construction
  line L2895 (-67.077, 4.3229) -> (-67.2288, 4.2639) construction
  line L2896 (-67.2288, 4.2639) -> (-67.3804, 4.2039) construction
  line L2897 (-67.3804, 4.2039) -> (-67.532, 4.143) construction
  line L2898 (-67.532, 4.143) -> (-67.6833, 4.0812) construction
  line L2899 (-67.6833, 4.0812) -> (-67.8345, 4.0185) construction
  line L2900 (-67.8345, 4.0185) -> (-67.9856, 3.9548) construction
  line L2901 (-67.9856, 3.9548) -> (-68.1365, 3.8903) construction
  line L2902 (-68.1365, 3.8903) -> (-68.2872, 3.8249) construction
  line L2903 (-68.2872, 3.8249) -> (-68.4378, 3.7585) construction
  line L2904 (-68.4378, 3.7585) -> (-68.5882, 3.6913) construction
  line L2905 (-68.5882, 3.6913) -> (-68.7384, 3.6233) construction
  line L2906 (-68.7384, 3.6233) -> (-68.8885, 3.5543) construction
  line L2907 (-68.8885, 3.5543) -> (-69.0384, 3.4846) construction
  line L2908 (-69.0384, 3.4846) -> (-69.1881, 3.4139) construction
  line L2909 (-69.1881, 3.4139) -> (-69.3376, 3.3425) construction
  line L2910 (-69.3376, 3.3425) -> (-69.487, 3.2701) construction
  line L2911 (-69.487, 3.2701) -> (-69.6362, 3.197) construction
  line L2912 (-69.6362, 3.197) -> (-69.7852, 3.123) construction
  line L2913 (-69.7852, 3.123) -> (-69.934, 3.0482) construction
  line L2914 (-69.934, 3.0482) -> (-70.0826, 2.9726) construction
  line L2915 (-70.0826, 2.9726) -> (-70.2311, 2.8962) construction
  line L2916 (-70.2311, 2.8962) -> (-70.3793, 2.819) construction
  line L2917 (-70.3793, 2.819) -> (-70.5274, 2.741) construction
  line L2918 (-70.5274, 2.741) -> (-70.6752, 2.6622) construction
  line L2919 (-70.6752, 2.6622) -> (-70.8229, 2.5826) construction
  line L2920 (-70.8229, 2.5826) -> (-70.9703, 2.5023) construction
  line L2921 (-70.9703, 2.5023) -> (-71.1176, 2.4211) construction
  line L2922 (-71.1176, 2.4211) -> (-71.2352, 2.3556) construction
  line L2923 (-71.2352, 2.3556) -> (-71.3234, 2.3061) construction
  line L2924 (-71.3234, 2.3061) -> (-71.3821, 2.2729) construction
  line L2925 (-71.3821, 2.2729) -> (-71.4115, 2.2563) construction
  line L2926 (-5.6951, -60.7685) -> (-5.6979, -60.7993) construction
  line L2927 (-5.6979, -60.7993) -> (-5.7029, -60.8609) construction
  line L2928 (-5.7029, -60.8609) -> (-5.7078, -60.9533) construction
  line L2929 (-5.7078, -60.9533) -> (-5.7097, -61.0766) construction
  line L2930 (-5.7097, -61.0766) -> (-5.7056, -61.231) construction
  line L2931 (-5.7056, -61.231) -> (-5.6969, -61.3856) construction
  line L2932 (-5.6969, -61.3856) -> (-5.6854, -61.5403) construction
  line L2933 (-5.6854, -61.5403) -> (-5.6723, -61.695) construction
  line L2934 (-5.6723, -61.695) -> (-5.6583, -61.8498) construction
  line L2935 (-5.6583, -61.8498) -> (-5.6431, -62.0045) construction
  line L2936 (-5.6431, -62.0045) -> (-5.6265, -62.1593) construction
  line L2937 (-5.6265, -62.1593) -> (-5.608, -62.314) construction
  line L2938 (-5.608, -62.314) -> (-5.5871, -62.4688) construction
  line L2939 (-5.5871, -62.4688) -> (-5.5641, -62.6235) construction
  line L2940 (-5.5641, -62.6235) -> (-5.539, -62.7782) construction
  line L2941 (-5.539, -62.7782) -> (-5.5121, -62.9329) construction
  line L2942 (-5.5121, -62.9329) -> (-5.4838, -63.0875) construction
  line L2943 (-5.4838, -63.0875) -> (-5.4542, -63.2421) construction
  line L2944 (-5.4542, -63.2421) -> (-5.4233, -63.3966) construction
  line L2945 (-5.4233, -63.3966) -> (-5.3913, -63.5511) construction
  line L2946 (-5.3913, -63.5511) -> (-5.3579, -63.7055) construction
  line L2947 (-5.3579, -63.7055) -> (-5.3232, -63.8598) construction
  line L2948 (-5.3232, -63.8598) -> (-5.2871, -64.014) construction
  line L2949 (-5.2871, -64.014) -> (-5.2497, -64.1682) construction